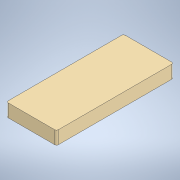
# Autodesk Inventor part: Controlador 1
Saved by Autodesk Inventor 2021.4 (Build 254397000, 397)
## iProperties
Created: 2022-11-18
Part Number: Controlador 1
Material: Genérico
Document SubType Name: Modeling
Designer: crist
Density: 1 g/cm^3
Appearance: Valor por defecto
Author: crist
Autodesk Inventor part; units mm, degrees
ref_plane "YZ Plane" through (0, 0, 0) normal (1, 0, 0) x (0, 1, 0)
ref_plane "XZ Plane" through (0, 0, 0) normal (0, 1, 0) x (-1, 0, 0)
ref_plane "XY Plane" through (0, 0, 0) normal (0, 0, 1) x (1, 0, 0)
sketch "Boceto1" plane through (0, 0, 0) normal (0, 1, 0) x (-1, 0, 0)
  line L0 (1, 0) -> (26, 0)
  line L1 (27, -1) -> (27, -62)
  line L2 (26, -63) -> (1, -63)
  line L3 (0, -62) -> (0, -1)
  arc A0 (26, -63) -> (27, -62) centre (26, -62) ccw
  arc A1 (27, -1) -> (26, 0) centre (26, -1) ccw
  arc A2 (1, 0) -> (0, -1) centre (1, -1) ccw
  arc A3 (0, -62) -> (1, -63) centre (1, -62) ccw
  point P0 (0, 0)
  point P1 (27, -63)
  point P2 (27, 0)
  point P3 (0, -63)
  dimension "d0" = 63
  dimension "d1" = 27
  dimension "d2" = 1
  constraints: 8 end point, 8 point on circle, 8 point on line, 8 tangent, 4 centre point, 3 equal radius, 2 parallel, 1 horizontal, 1 perpendicular
  measures "d0" distance of point (27, 0) point (27, -63)
  measures "d1" distance of point (27, -63) point (0, -63)
  measures "d2" radius of A0
extrude "Extrusión1" add sketch "Boceto1" along normal blind 7
sketch "Boceto2" plane through (0, 7, 0) normal (0, 1, 0) x (1, 0, 0)
  line L0 (-27, 62) -> (-27, 1) projected
  line L1 (-27, 62) -> (-27, 63.4862)
  line L2 (-25.9515, 63.0037) -> (-27.3185, 63.0037)
  line L3 (-27, 63.0037) -> (-22, 63)
  line L4 (-1, 63) -> (-26, 63) projected
  line L5 (-22, 63) -> (-22, 58)
  circle A0 centre (-22, 58) radius 1.5
  point P0 (0, 0)
  dimension "d5" = 5
  dimension "d7" = 5
  dimension "d8" = 3
  constraints: 8 end point, 3 point on line, 1 centre point, 1 coincident, 1 horizontal, 1 perpendicular, 1 vertical
  measures "d5" distance of L3.start L3.end
  measures "d7" distance of L3.end L5.end
  measures "d8" diameter of A0
sketch "Boceto3" plane through (0, 0, 0) normal (0, -1, 0) x (1, 0, 0)
  arc A0 (-27, -62) -> (-26, -63) centre (-26, -62) ccw projected
  line L0 (-26, -63) -> (-27.2127, -63)
  line L1 (-27, -62) -> (-27, -1) projected
  line L2 (-27, -61.713) -> (-27, -63.5495)
  line L3 (-27, -63) -> (-27, -58)
  line L4 (-27, -58) -> (-22, -58)
  circle A1 centre (-22, -58) radius 1.5
  point P0 (0, 0)
  dimension "d9" = 5
  dimension "d10" = 5
  dimension "d11" = 3
  constraints: 8 end point, 4 point on line, 2 perpendicular, 1 centre point, 1 coincident, 1 horizontal, 1 tangent
  measures "d9" distance of L3.start L3.end
  measures "d10" distance of L3.end L4.end
  measures "d11" diameter of A1
